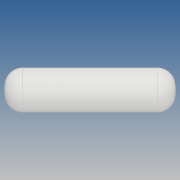
# Autodesk Inventor part: 轴
Saved by Autodesk Inventor 2019.1 (Build 231200000, 200)
## iProperties
Created: 2020-09-27
Part Number: 轴
Material: ABS 塑料
Document SubType Name: Modeling
Designer: 谢庆红冰
Density: 1.06 g/cm^3
Appearance: 平滑 - 白色
Company: 北京理工大学
Author: 谢庆红冰
## iProperties of the stored document 轴_bate_3D 打印.ipt
Created: 2020-09-29
Part Number: 轴_bate_3D 打印
Material: Generic
Document SubType Name: Modeling
Designer: 谢庆红冰
Density: 1 g/cm^3
Appearance: Default
Author: 谢庆红冰
Autodesk Inventor part; units mm, degrees
sketch "草图1" plane through (0, 0, 0) normal (0, 0, 1) x (1, 0, 0)
  line L0 (3.25, 4.75) -> (3.25, 2.25) projected
  line L1 (2.75, 2.75) -> (5.25, 2.75) projected
  arc A0 (3.25, 2.25) -> (4.75, 2.25) centre (4, 2.25) ccw projected
  line L2 (4.75, 2.25) -> (4.75, 4.75) projected
  arc A1 (5.25, 2.75) -> (5.25, 4.25) centre (5.25, 3.5) ccw projected
  line L3 (5.25, 4.25) -> (2.75, 4.25) projected
  line L4 (2.75, 2.75) -> (5.25, 2.75) projected
  arc A2 (2.75, 4.25) -> (2.75, 2.75) centre (2.75, 3.5) ccw projected
  arc A3 (4.75, 4.75) -> (3.25, 4.75) centre (4, 4.75) ccw projected
  circle A4 centre (4, 3.5) radius 2.5
  line L5 (2.75, 3.5) -> (5.25, 3.5)
  point P0 (0, 0)
  dimension "d7" = 5
  constraints: 2 end point, 1 centre point, 1 midpoint, 1 perpendicular
  measures "d7" diameter of A4
ref_plane "工作平面1" through (-7.5, 0, 7.5) normal (0, 0, 1) x (1, 0, 0)
ref_plane "工作平面2" through (7.5, 0, -7.5) normal (0, 0, -1) x (-1, 0, 0)
sketch "草图2" plane through (0, 0, 0) normal (0, 1, 0) x (-1, 0, 0)
  line L0 (1.1, -7.5) -> (-6.6, -7.5) construction
  line L1 (-6.6, 7.5) -> (1.1, 7.5) construction
  point P0 (0, 0)
  dimension "d0" = 15
  measures "d0" distance between parallel lines of L0 L1
extrude "拉伸1" add sketch "草图1" along normal mid plane 19 contours A3 L2 L3 L0 | L3 L2 L5 L0 | L0 L1 A2 L3 | L5 L2 L1 L0 | L3 A1 L1 L2 | L1 L2 A0 L0 | A4
fillet "圆角1" [suppressed]
fillet "圆角2" [suppressed]
fillet "圆角3" [suppressed]
sketch "草图3" plane through (0, 0, -9.5) normal (0, 0, -1) x (-1, 0, 0)
  arc A0 (-3.75, 4.75) -> (-2.75, 3.75) centre (-2.75, 4.75) ccw construction
  arc A1 (-3.75, 4.75) -> (-4.25, 4.75) centre (-4, 4.75) ccw construction
  arc A2 (-5.25, 3.75) -> (-4.25, 4.75) centre (-5.25, 4.75) ccw construction
  arc A3 (-5.25, 3.75) -> (-5.25, 3.25) centre (-5.25, 3.5) ccw construction
  arc A4 (-4.25, 2.25) -> (-5.25, 3.25) centre (-5.25, 2.25) ccw construction
  arc A5 (-4.25, 2.25) -> (-3.75, 2.25) centre (-4, 2.25) ccw construction
  arc A6 (-2.75, 3.25) -> (-3.75, 2.25) centre (-2.75, 2.25) ccw construction
  arc A7 (-2.75, 3.25) -> (-2.75, 3.75) centre (-2.75, 3.5) ccw construction
  line L0 (-4, 4.75) -> (-4, 2.25)
  point P0 (0, 0)
  point P1 (-4, 3.5)
  constraints: 2 end point, 1 midpoint, 1 vertical
sketch "草图4" plane through (0, 0, 9.5) normal (0, 0, 1) x (1, 0, 0)
  arc A0 (4.25, 4.75) -> (3.75, 4.75) centre (4, 4.75) ccw construction
  arc A1 (2.75, 3.75) -> (3.75, 4.75) centre (2.75, 4.75) ccw construction
  arc A2 (2.75, 3.75) -> (2.75, 3.25) centre (2.75, 3.5) ccw construction
  arc A3 (3.75, 2.25) -> (2.75, 3.25) centre (2.75, 2.25) ccw construction
  arc A4 (3.75, 2.25) -> (4.25, 2.25) centre (4, 2.25) ccw construction
  arc A5 (5.25, 3.25) -> (4.25, 2.25) centre (5.25, 2.25) ccw construction
  arc A6 (5.25, 3.25) -> (5.25, 3.75) centre (5.25, 3.5) ccw construction
  arc A7 (4.25, 4.75) -> (5.25, 3.75) centre (5.25, 4.75) ccw construction
  line L0 (5.25, 3.5) -> (2.75, 3.5)
  point P0 (0, 0)
  point P1 (4, 3.5)
  constraints: 2 end point, 1 horizontal, 1 midpoint
ref_plane "工作平面3" through (0, 0, 0) normal (0, 0, 1) x (1, 0, 0)
fillet "圆角4" radius 2 2 edges at (1.5, 3.5, 9.5) (1.5, 3.5, -9.5)
